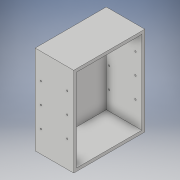
# Autodesk Inventor part: Cart Box
Saved by Autodesk Inventor 2018 (Build 220112000, 112)
## iProperties
Created: 2018-12-10
Part Number: Cart Box
Material: Generic
Document SubType Name: Modeling
Designer: Gabriel
Density: 1 g/cm^3
Appearance: Default
Author: Gabriel
Autodesk Inventor part; units mm, degrees
ref_plane "YZ Plane" through (0, 0, 0) normal (1, 0, 0) x (0, 1, 0)
ref_plane "XZ Plane" through (0, 0, 0) normal (0, 1, 0) x (-1, 0, 0)
ref_plane "XY Plane" through (0, 0, 0) normal (0, 0, 1) x (1, 0, 0)
sketch "Sketch1" plane through (0, 0, 0) normal (1, 0, 0) x (0, 1, 0)
  line L0 (6.7738, 9.1186) -> (-755.2262, 9.1186)
  line L1 (-755.2262, 9.1186) -> (-755.2262, -600.4814)
  line L2 (-755.2262, -600.4814) -> (6.7738, -600.4814)
  line L3 (6.7738, -600.4814) -> (6.7738, 9.1186)
  line L4 (-18.6262, -16.2814) -> (-729.8262, -16.2814)
  line L5 (-729.8262, -16.2814) -> (-729.8262, -575.0814)
  line L6 (-729.8262, -575.0814) -> (-18.6262, -575.0814)
  line L7 (-18.6262, -575.0814) -> (-18.6262, -16.2814)
  point P0 (0, 0)
  dimension "d0" = 762
  dimension "d1" = 609.6
  dimension "d2" = 25.4
  constraints: 16 end point, 4 parallel, 2 perpendicular, 1 horizontal, 3 other
  measures "d0" distance of L2.end L1.end
  measures "d1" distance of L1.end L0.end
  measures "d2" distance between parallel lines of L3 L7
extrude "Extrusion3" add sketch "Sketch1" along normal blind 304.8
sketch "Sketch4" plane through (0, 0, 0) normal (-1, 0, 0) x (0, 0, 1)
  line L0 (9.1186, 6.7738) -> (9.1186, -755.2262) projected
  line L1 (9.1186, -755.2262) -> (-600.4814, -755.2262) projected
  line L2 (9.1186, 6.7738) -> (-600.4814, 6.7738)
  line L3 (-600.4814, 6.7738) -> (-600.4814, -755.2262)
  line L4 (-600.4814, -755.2262) -> (9.1186, -755.2262)
  line L5 (9.1186, -755.2262) -> (9.1186, 6.7738)
  point P0 (0, 0)
  constraints: 8 end point, 2 parallel, 1 horizontal, 1 perpendicular
extrude "Extrusion4" add sketch "Sketch4" along normal blind 25.4
sketch "Sketch5" plane through (304.8, -755.2262, -600.4814) normal (0, 0, -1) x (-1, 0, 0)
  line L0 (0, 762) -> (330.2, 762) projected
  line L1 (330.2, 762) -> (330.2, 533.4)
  line L2 (330.2, 762) -> (330.2, 0) projected
  line L3 (330.2, 533.4) -> (330.2, 355.6)
  line L4 (330.2, 355.6) -> (330.2, 177.8)
  line L5 (330.2, 533.4) -> (55.0447, 581.9173)
  line L6 (330.2, 533.4) -> (609.6, 533.4) construction
  line L7 (330.2, 355.6) -> (55.0447, 404.1173)
  line L8 (330.2, 355.6) -> (609.6, 355.6) construction
  line L9 (330.2, 177.8) -> (55.0447, 226.3173)
  line L10 (330.2, 177.8) -> (609.6, 177.8) construction
  circle A0 centre (55.0447, 404.1173) radius 6.35
  circle A1 centre (55.0447, 581.9173) radius 6.35
  circle A2 centre (55.0447, 226.3173) radius 6.35
  line L11 (330.2, 533.4) -> (280.1718, 542.2213)
  line L12 (330.2, 533.4) -> (381, 533.4) construction
  line L13 (330.2, 355.6) -> (280.1718, 364.4213)
  line L14 (330.2, 355.6) -> (381, 355.6) construction
  line L15 (330.2, 177.8) -> (280.1718, 186.6213)
  line L16 (330.2, 177.8) -> (381, 177.8) construction
  circle A3 centre (280.1718, 542.2213) radius 6.35
  circle A4 centre (280.1718, 364.4213) radius 6.35
  circle A5 centre (280.1718, 186.6213) radius 6.35
  point P0 (304.8, 755.2262)
  dimension "d16" = 177.8
  dimension "d17" = 177.8
  dimension "d26" = 279.4
  dimension "d27" = 170
  dimension "d28" = 279.4
  dimension "d29" = 170
  dimension "d30" = 279.4
  dimension "d31" = 170
  dimension "d32" = 12.7
  dimension "d33" = 12.7
  dimension "d34" = 12.7
  dimension "d35" = 50.8
  dimension "d36" = 170
  dimension "d37" = 50.8
  dimension "d38" = 170
  dimension "d39" = 50.8
  dimension "d40" = 170
  dimension "d41" = 12.7
  dimension "d42" = 12.7
  dimension "d43" = 12.7
  constraints: 30 end point, 6 centre point, 6 coincident, 6 equal length, 6 horizontal, 3 parallel, 3 point on line
  measures "d16" distance of L1.end L3.end
  measures "d17" distance of L3.end L4.end
  measures "d26" distance of L1.end L5.end
  measures "d27" angle of L6 L5
  measures "d28" distance of L3.end L7.end
  measures "d29" angle of L8 L7
  measures "d30" distance of L4.end L9.end
  measures "d31" angle of L10 L9
  measures "d32" diameter of A0
  measures "d33" diameter of A1
  measures "d34" diameter of A2
  measures "d35" distance of L1.end L11.end
  measures "d36" angle of L12 L11
  measures "d37" distance of L3.end L13.end
  measures "d38" angle of L14 L13
  measures "d39" distance of L4.end L15.end
  measures "d40" angle of L16 L15
  measures "d41" diameter of A3
  measures "d42" diameter of A4
  measures "d43" diameter of A5
extrude "Extrusion6" cut sketch "Sketch5" against normal blind 914.4
body "Solid1"
